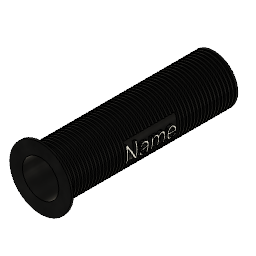
HandleBar (Autodesk Fusion 360 design; units mm, degrees)
part number: 2026-06-08-19-54-29-010
Autodesk Fusion 360 part; units mm, degrees
note: some values were not read from the file. Set by a fixed rule: which sketch regions a step uses.
sketch "Sketch1" plane through (0, 0, 0) normal (0, 1, 0) x (1, 0, 0)
  circle A0 centre (0, 0) radius 15
  dimension "d1" = 30
  constraint coincident A0.centre origin
  measures "d1" diameter of A0
extrude "Extrude1" add sketch "Sketch1" along normal blind 125 makes body 1
sketch "Sketch2" plane through (0, 0, 0) normal (1, 0, 0) x (0, 1, 0)
sketch "Sketch4" plane through (0, 0, 0) normal (1, 0, 0) x (0, 1, 0)
  line L0 (0, -15) -> (125, -15) construction
  line L1 (125, -15) -> (125, 15) construction
  line L2 (125, 15) -> (0, 15) construction
  line L3 (0, 15) -> (0, -15) construction
  point P0 (0, 15)
  point P1 (0, -15)
  point P2 (125, 15)
  point P3 (125, -15)
  dimension "d4" = 10
  text T0 "Name" font "Arial" height 10 align centre middle in box 125 x 30 at (0, -15) x (1, 0) y (0, 1) spacing 1
  constraint coincident P0
  constraint coincident P2
  constraint coincident P3
shell "Shell1" thickness 2 removed faces 1 at (0.9463, 0, 5.6032) on bodies 1
emboss "Emboss1" depth 2 profiles "Sketch4" section 1 text T0 onto face at (14.9814, 83.3333, 0.7477) on bodies 1 bodies 1
sketch "Sketch5" plane through (0, 0, 0) normal (0, 1, 0) x (1, 0, 0)
  circle A0 centre (0, 0) radius 15
  circle A1 centre (0, 0) radius 17
  line L0 (14.9097, -8.1671) -> (13.1338, -7.2458)
  line L1 (14.6966, 8.5446) -> (12.9821, 7.5143)
  point P0 (16.0643, -5.5623)
  point P1 (16.0643, 5.5623)
  dimension "d10" = 2
  constraint coincident A1 L0.start
  constraint coincident A0 L0.end
  constraint coincident A1 L1.start
  constraint coincident A0 L1.end
extrude "Extrude2" add sketch "Sketch5" along normal blind 1.5 separate body contours A0 A1 L0 L1 | A0 A1 L0 L1 makes body 2
pattern_linear "R-Pattern1" count 50 spacing 2.5 along (0, 1, 0) of bodies 2 makes body 3 at (13.8689, 2.5, 8.554) makes body 4 at (13.8689, 5, 8.554) makes body 5 at (13.8689, 7.5, 8.554) makes body 6 at (13.8689, 10, 8.554) makes body 7 at (13.8689, 12.5, 8.554) makes body 8 at (13.8689, 15, 8.554) makes body 9 at (13.8689, 17.5, 8.554) makes body 10 at (13.8689, 20, 8.554) makes body 11 at (13.8689, 22.5, 8.554) makes body 12 at (13.8689, 25, 8.554) makes body 13 at (13.8689, 27.5, 8.554) makes body 14 at (13.8689, 30, 8.554) makes body 15 at (13.8689, 32.5, 8.554) makes body 16 at (13.8689, 35, 8.554) makes body 17 at (13.8689, 37.5, 8.554) makes body 18 at (13.8689, 40, 8.554) makes body 19 at (13.8689, 42.5, 8.554) makes body 20 at (13.8689, 45, 8.554) makes body 21 at (13.8689, 47.5, 8.554) makes body 22 at (13.8689, 50, 8.554) makes body 23 at (13.8689, 52.5, 8.554) makes body 24 at (13.8689, 55, 8.554) makes body 25 at (13.8689, 57.5, 8.554) makes body 26 at (13.8689, 60, 8.554) makes body 27 at (13.8689, 62.5, 8.554) makes body 28 at (13.8689, 65, 8.554) makes body 29 at (13.8689, 67.5, 8.554) makes body 30 at (13.8689, 70, 8.554) makes body 31 at (13.8689, 72.5, 8.554) makes body 32 at (13.8689, 75, 8.554) makes body 33 at (13.8689, 77.5, 8.554) makes body 34 at (13.8689, 80, 8.554) makes body 35 at (13.8689, 82.5, 8.554) makes body 36 at (13.8689, 85, 8.554) makes body 37 at (13.8689, 87.5, 8.554) makes body 38 at (13.8689, 90, 8.554) makes body 39 at (13.8689, 92.5, 8.554) makes body 40 at (13.8689, 95, 8.554) makes body 41 at (13.8689, 97.5, 8.554) makes body 42 at (13.8689, 100, 8.554) makes body 43 at (13.8689, 102.5, 8.554) makes body 44 at (13.8689, 105, 8.554) makes body 45 at (13.8689, 107.5, 8.554) makes body 46 at (13.8689, 110, 8.554) makes body 47 at (13.8689, 112.5, 8.554) makes body 48 at (13.8689, 115, 8.554) makes body 49 at (13.8689, 117.5, 8.554) makes body 50 at (13.8689, 120, 8.554) makes body 51 at (13.8689, 122.5, 8.554)
extrude "Extrude3" cut sketch "Sketch5" along normal up to surface (82.5 mm away) contours A0 A1 L0 L1 picked at (14.4566, 7.5334) bodies 20 21 22 23 24 25 26 27 28 29 30 31 32 33 34
combine "Combine1" operation add target body 1 tool bodies 2 3 4 5 6 7 8 9 10 11 12 13 14 15 16 17 18 19 20 21 22 23 24 25 26 27 28 29 30 31 32 33 34 35 36 37 38 39 40 41 42 43 44 45 46 47 48 49 50 51
sketch "Sketch7" plane through (0, 0, 0) normal (0, -1, 0) x (1, 0, 0)
  circle A0 centre (0, 0) radius 17
  circle A1 centre (0, 0) radius 13
  circle A2 centre (0, 0) radius 22
  dimension "d20" = 5
extrude "Extrude4" add sketch "Sketch7" against normal blind 1.5 contours A2 bodies 1
equation "d5 = 'Name'"
